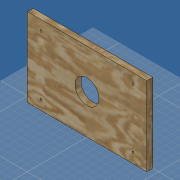
# Autodesk Inventor part: Korpus_Einbau_Basis
Saved by Autodesk Inventor 2019 (Build 230136000, 136)
## iProperties
Created: 2020-08-04
Part Number: Korpus_Einbau_Basis
Material: Generisch
Document SubType Name: Modeling
Designer: Stefan
Mass: 1494.75 g
Surface Area: 1934.26 cm^2
Volume: 1494.75 cm^3
Density: 1 g/cm^3
Appearance: Sperrholz - verwittert
Author: Stefan
Autodesk Inventor part; units mm, degrees
ref_plane "YZ Plane" through (0, 0, 0) normal (1, 0, 0) x (0, 1, 0)
ref_plane "XZ Plane" through (0, 0, 0) normal (0, 1, 0) x (-1, 0, 0)
ref_plane "XY Plane" through (0, 0, 0) normal (0, 0, 1) x (1, 0, 0)
sketch "Skizze1" plane through (0, 0, 0) normal (0, 0, 1) x (1, 0, 0)
  line L0 (-182, -120) -> (182, -120)
  line L1 (182, -120) -> (182, 120)
  line L2 (182, 120) -> (-182, 120)
  line L3 (-182, 120) -> (-182, -120)
  line L4 (-182, -120) -> (182, 120) construction
  line L5 (182, -120) -> (-182, 120) construction
  circle A0 centre (0, 0) radius 36.5
  line L6 (-140, -90) -> (140, -90)
  line L7 (140, -90) -> (140, 90)
  line L8 (140, 90) -> (-140, 90)
  line L9 (-140, 90) -> (-140, -90)
  line L10 (-140, -90) -> (140, 90) construction
  line L11 (140, -90) -> (-140, 90) construction
  circle A1 centre (-140, 90) radius 3.25
  circle A2 centre (140, 90) radius 3.25
  circle A3 centre (140, -90) radius 3.25
  circle A4 centre (-140, -90) radius 3.25
  point P0 (0, 0)
  point P1 (0, 0)
  point P2 (0, 0)
  dimension "d0" = 364
  dimension "d1" = 240
  dimension "d5" = 73
  dimension "d6" = 280
  dimension "d7" = 180
  dimension "d8" = 6.5
  constraints: 24 end point, 7 midpoint, 5 centre point, 5 coincident, 4 parallel, 3 equal radius, 2 horizontal, 2 perpendicular
  measures "d0" distance of L1.end L2.end
  measures "d1" distance of L2.end L0.start
  measures "d5" diameter of A0
  measures "d6" distance of L8.end L7.end
  measures "d7" distance of L7.end L6.end
  measures "d8" diameter of A1
extrude "Extrusion1" add sketch "Skizze1" along normal blind 18 contours L3 L2 L1 L0 | L9 A4 L6 | L6 A4 L9 | A4 L9 A1 L8 A2 L7 A3 L6 | A3 L7 L6 | L6 L7 A3 | A1 L8 L9 | L9 L8 A1 | A2 L8 L7 | L7 L8 A2
extrude "Extrusion2" cut sketch "Skizze1" along normal through all contours L9 A4 L6 | L6 A4 L9 | A3 L7 L6 | L6 L7 A3 | A1 L8 L9 | L9 L8 A1 | A2 L8 L7 | L7 L8 A2
equation "\"d0\" = case_width - 2 * case_thickness"
equation "\"d1\" = inner_depth - inner_thickness"
equation "\"d2\" = case_thickness"
equation "\"kg_thickness\" = 4.9"
equation "\"ht_thickness\" = 1.9"
equation "\"case_thickness\" = 18"
equation "\"inner_thickness\" = 15"
equation "\"gap_fit\" = 0.1"
equation "\"gap_slide\" = 0.2"
equation "\"gap_air\" = 1"
equation "\"bore_diameter\" = 73"
equation "\"mdf_thickness\" = 6"
equation "\"tape_width\" = 15"
equation "\"tape_thickness\" = 3"
equation "\"inner_depth\" = 255"
equation "\"case_width\" = 400"
